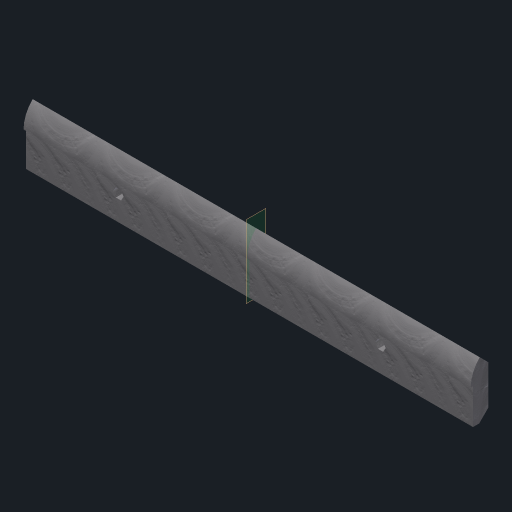
# Autodesk Inventor part: ESQUINA_REDONDEADA_R20
Saved by Autodesk Inventor 2024.3 (Build 283343000, 343)
## iProperties
Created: 2024-05-19
Part Number: ESQUINA_REDONDEADA_R20
Material: Steel, Mild, Welded
Document SubType Name: Modeling
Designer: Niler
Density: 7.85 g/cm^3
Appearance: Weld - Steel Mild
Author: Niler
Autodesk Inventor part; units mm, degrees
ref_plane "YZ Plane" through (0, 0, 0) normal (1, 0, 0) x (0, 1, 0)
ref_plane "XZ Plane" through (0, 0, 0) normal (0, 1, 0) x (-1, 0, 0)
ref_plane "XY Plane" through (0, 0, 0) normal (0, 0, 1) x (1, 0, 0)
sketch "Sketch1" plane through (0, 0, 0) normal (1, 0, 0) x (0, 1, 0)
  circle A0 centre (0, 0) radius 20
  line L0 (8.5, 8.5) -> (-16.9, 8.5)
  line L1 (8.5, 8.5) -> (8.5, -16.9)
  line L2 (0, 0) -> (0, 20)
  line L3 (0, 20) -> (-60.9241, 20)
  line L4 (-60.9241, 20) -> (-60.9241, 18.5)
  line L5 (-60.9241, 18.5) -> (0, 18.5)
  line L6 (0, 18.5) -> (0, 20)
  line L7 (0, 0) -> (14.1421, 14.1421)
  line L8 (0, 0) -> (20, 0)
  line L9 (-16.9, 8.5) -> (-16.9, 18.5)
  line L10 (-16.9, 8.5) -> (-22.9, 14.5)
  line L11 (-22.9, 14.5) -> (-22.9, 18.5)
  line L12 (12.3744, 12.3744) -> (12.1502, 13.2109)
  line L13 (11.3137, 13.435) -> (9.2071, 11.3284)
  line L14 (9.4313, 10.4919) -> (10.2678, 10.2678)
  line L15 (8.5, 8.5) -> (8.5, -16.9)
  line L16 (20, 0) -> (20, -60.9241)
  line L17 (20, -60.9241) -> (18.5, -60.9241)
  line L18 (18.5, -60.9241) -> (18.5, 0)
  line L19 (8.5, -16.9) -> (18.5, -16.9)
  line L20 (8.5, -16.9) -> (14.5, -22.9)
  line L21 (14.5, -22.9) -> (18.5, -22.9)
  arc A1 (9.2071, 11.3284) -> (9.4313, 10.4919) centre (9.5607, 10.9749) ccw
  arc A2 (12.1502, 13.2109) -> (11.3137, 13.435) centre (11.6673, 13.0815) ccw
  line L22 (10.4311, 10.4311) -> (9.483, 10.6851)
  arc A3 (9.3485, 11.187) -> (9.483, 10.6851) centre (9.5607, 10.9749) ccw
  line L23 (9.3485, 11.187) -> (11.4551, 13.2936)
  arc A4 (11.957, 13.1591) -> (11.4551, 13.2936) centre (11.6673, 13.0815) ccw
  line L24 (11.957, 13.1591) -> (12.2111, 12.2111)
  point P0 (0, 8.5)
  point P1 (-17.7041, 9.3041)
  point P2 (-16.9, 10.6953)
  dimension "d0" = 40
  dimension "d1" = 25.4
  dimension "d2" = 1.5
  dimension "d4" = 45
  dimension "d6" = 45
  dimension "d7" = 4
  dimension "d8" = 10
  dimension "d10" = 2.5
  dimension "d11" = 2.5
  dimension "d12" = 60
  dimension "d13" = 1.5
  dimension "d15" = 0.5
  dimension "d16" = 0.2
  constraints: 50 end point, 11 point on circle, 10 point on line, 6 symmetric about line, 5 centre point, 4 perpendicular, 4 tangent, 3 parallel, 2 equal length, 2 horizontal, 2 vertical, 1 coincident, 1 equal radius, 1 vertical alignment, 4 other
  measures "d0" diameter of A0
  measures "d1" distance of L0.start L1.end
  measures "d2" distance of L4.end L3.end
  measures "d4" angle of L2 L7
  measures "d6" angle of L9 L10
  measures "d7" distance of L10.end L11.end
  measures "d8" distance between parallel lines of L0 L5
  measures "d10" distance of L7.end L12.start
  measures "d11" distance of L0.start L14.end
  measures "d12" angle of L7 L12
  measures "d13" distance between parallel lines of L7 L13
  measures "d15" radius of A1
  measures "d16" distance between parallel lines of L13 L23
extrude "Extrusion1" add sketch "Sketch1" along normal blind 290 contours L7 L12 A2 L13 A1 L14 L0 L2 A0 | L7 L24 A4 L23 A3 L22 L14 A1 L13 A2 L12 | L5 L2 L0 L9 A0 | A0 L9 L5 | L7 L22 A3 L23 A4 L24 | L9 L10 A0 | A0 L10 L11 L5 L9
sketch "Sketch2" plane through (0, -22.9, 18.5) normal (0, 0, 1) x (1, 0, 0)
  line L0 (0, 22.9) -> (0, 0) projected
  line L1 (0, 0) -> (290, 0) projected
  line L2 (290, 22.9) -> (290, 0) projected
  line L3 (0, 22.9) -> (290, 22.9) projected
  line L4 (58.3257, 13.1) -> (56.6514, 16)
  line L5 (56.6514, 16) -> (58.3257, 18.9)
  line L6 (58.3257, 18.9) -> (61.6743, 18.9)
  line L7 (61.6743, 18.9) -> (63.3486, 16)
  line L8 (63.3486, 16) -> (61.6743, 13.1)
  line L9 (61.6743, 13.1) -> (58.3257, 13.1)
  line L10 (0, 6) -> (290, 6) projected
  circle A0 centre (60, 16) radius 1.65
  dimension "d20" = 10
  dimension "d21" = 5.8
  dimension "d22" = 60
  dimension "d25" = 3.3
  constraints: 12 end point, 1 centre point, 1 coincident, 1 horizontal alignment, 13 other
  measures "d20" distance from line of L10 point (60, 16)
  measures "d21" distance between parallel lines of L9 L6
  measures "d22" distance from line of point (60, 16) L0
  measures "d25" diameter of A0
extrude "Extrusion2" cut sketch "Sketch2" against normal blind 6 contours L4 L5 L6 L7 L8 L9 | A0
extrude "Extrusion3" cut sketch "Sketch2" against normal through all contours A0
sketch "Sketch3" plane through (0, -22.9, 18.5) normal (0, 0, 1) x (1, 0, 0)
  line L0 (0, 37.0421) -> (290, 37.0421) projected
  line L1 (0, 0) -> (290, 0) projected
  line L2 (0, 22.9) -> (0, 0) projected
  line L3 (0, 22.9) -> (0, 37.0421) projected
  line L4 (2.4384, 37.0421) -> (17.8575, 0)
  line L5 (0, 0) -> (290, 0) projected
  line L6 (2.4384, 37.0421) -> (0, 42.9) projected
  point P0 (0, 26.9698)
  dimension "d28" = 112.6
  constraints: 2 end point, 1 point on line
  measures "d28" angle of L4 L0
ref_plane "Work Plane1" through (145, 0, 0) normal (-1, 0, 0) x (0, 0, 1)
mirror "Mirror1" about plane through (145, 0, 0) normal (-1, 0, 0) of "Extrusion2", "Extrusion3"
body "Solid1"
